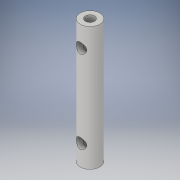
# Autodesk Inventor part: ConnectorRod
Saved by Autodesk Inventor 2017 (Build 210142000, 142)
## iProperties
Created: 2016-06-07
Part Number: ConnectorRod
Material: Generic
Document SubType Name: Modeling
Designer: steele
Density: 1 g/cm^3
Appearance: Default
Author: steele
Autodesk Inventor part; units mm, degrees
ref_plane "YZ Plane" through (0, 0, 0) normal (1, 0, 0) x (0, 1, 0)
ref_plane "XZ Plane" through (0, 0, 0) normal (0, 1, 0) x (-1, 0, 0)
sketch "Sketch1" plane through (0, 0, 0) normal (0, 1, 0) x (-1, 0, 0)
  circle A0 centre (0, 0) radius 6.0325
  circle A1 centre (0, 0) radius 2.8575
  dimension "d0" = 12.065
  dimension "d1" = 5.715
  constraints: 2 centre point, 2 coincident
  measures "d0" diameter of A0
  measures "d1" diameter of A1
extrude "Extrusion1" add sketch "Sketch1" along normal mid plane 76.2
ref_plane "Work Plane1" through (0, 0, 6.0325) normal (0, 0, 1) x (1, 0, 0)
sketch "Sketch2" plane through (0, 0, 6.0325) normal (0, 0, 1) x (1, 0, 0)
  line L0 (6.0325, 38.1) -> (-6.0325, 38.1) projected
  line L1 (-6.0325, -38.1) -> (6.0325, -38.1) projected
  point P0 (0, 0)
  point P1 (0, 25.4)
  point P2 (0, -25.4)
  dimension "d4" = 12.7
  dimension "d5" = 12.7
  measures "d4" distance from line of point (0, 25.4) L0
  measures "d5" distance from line of point (0, -25.4) L1
hole "Hole1" at (0, 25.4, 6.0325) at (0, -25.4, 6.0325) direction (0, 0, -1) diameter 6.35 end through all
body "Solid1"
